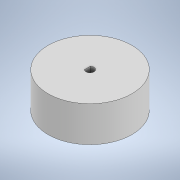
# Autodesk Inventor part: Kolo_Pololu1127
Saved by Autodesk Inventor 2021 (Build 250183000, 183)
## iProperties
Created: 2021-03-30
Part Number: Kolo_Pololu1127
Material: Ogólny
Document SubType Name: Modeling
Designer: jakub
Density: 1 g/cm^3
Appearance: Domyślna
Author: jakub
Autodesk Inventor part; units mm, degrees
ref_plane "YZ Plane" through (0, 0, 0) normal (1, 0, 0) x (0, 1, 0)
ref_plane "XZ Plane" through (0, 0, 0) normal (0, 1, 0) x (-1, 0, 0)
ref_plane "XY Plane" through (0, 0, 0) normal (0, 0, 1) x (1, 0, 0)
sketch "Szkic1" plane through (0, 0, 0) normal (0, 1, 0) x (-1, 0, 0)
  circle A0 centre (0, 0) radius 15.6
  dimension "d0" = 31.2
  constraints: 1 centre point, 1 coincident
  measures "d0" diameter of A0
extrude "Wyciągnięcie proste1" add sketch "Szkic1" along normal blind 13.2
sketch "Szkic3" plane through (0, 13.2, 0) normal (0, 1, 0) x (1, 0, 0)
  arc A0 (-1, -1.118) -> (-1, 1.118) centre (0, 0) ccw
  line L0 (-1, 1.118) -> (-1, -1.118)
  constraints: 2 end point, 2 point on circle, 1 centre point
extrude "Wyciągnięcie proste2" cut sketch "Szkic3" against normal blind 13.2
